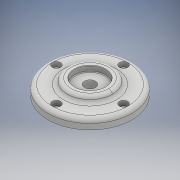
# Autodesk Inventor part: 도면2-3번
Saved by Autodesk Inventor 2018.3 (Build 223284000, 284)
## iProperties
Created: 2019-10-10
Part Number: 도면2-3번
Material: 일반
Document SubType Name: Modeling
Designer: MyTool
Density: 1 g/cm^3
Appearance: 기본값
Author: MyTool
Autodesk Inventor part; units mm, degrees
ref_plane "YZ Plane" through (0, 0, 0) normal (1, 0, 0) x (0, 1, 0)
ref_plane "XZ Plane" through (0, 0, 0) normal (0, 1, 0) x (-1, 0, 0)
ref_plane "XY Plane" through (0, 0, 0) normal (0, 0, 1) x (1, 0, 0)
sketch "스케치4" plane through (0, 0, 0) normal (0, 0, 1) x (1, 0, 0)
  circle A0 centre (0, 0) radius 30
  dimension "d28" = 60
  constraints: 1 centre point, 1 coincident
  measures "d28" diameter of A0
extrude "돌출4" add sketch "스케치4" along normal blind 7
sketch "스케치5" plane through (0, 0, 7) normal (0, 0, 1) x (1, 0, 0)
  circle A0 centre (0, 0) radius 16
  dimension "d31" = 32
  constraints: 1 centre point, 1 coincident
  measures "d31" diameter of A0
extrude "돌출5" add sketch "스케치5" along normal blind 4
sketch "스케치6" plane through (0, 0, 0) normal (0, 0, -1) x (-1, 0, 0)
  circle A0 centre (0, 0) radius 17.5
  dimension "d34" = 35
  constraints: 1 centre point, 1 coincident
  measures "d34" diameter of A0
extrude "돌출6" add sketch "스케치6" along normal blind 4
sketch "스케치8" plane through (0, 0, 11) normal (0, 0, 1) x (1, 0, 0)
  circle A0 centre (0, 0) radius 11
  dimension "d41" = 22
  constraints: 1 centre point, 1 coincident
  measures "d41" diameter of A0
extrude "돌출8" cut sketch "스케치8" against normal blind 4
sketch "스케치9" plane through (0, 0, -4) normal (0, 0, -1) x (-1, 0, 0)
  circle A0 centre (0, 0) radius 9.5
  dimension "d44" = 19
  constraints: 1 centre point, 1 coincident
  measures "d44" diameter of A0
extrude "돌출9" cut sketch "스케치9" against normal blind 4
sketch "스케치11" plane through (0, 0, 7) normal (0, 0, 1) x (1, 0, 0)
  circle A0 centre (0, 0) radius 4
  dimension "d49" = 8
  constraints: 1 centre point, 1 coincident
  measures "d49" diameter of A0
extrude "돌출10" cut sketch "스케치11" against normal up to next
sketch "스케치12" plane through (0, 0, 7) normal (0, 0, 1) x (1, 0, 0)
  circle A0 centre (0, 24) radius 3
  point P0 (0, 0)
  dimension "d61" = 6
  dimension "d62" = 24
  constraints: 1 centre point
  measures "d61" diameter of A0
  measures "d62" distance of point (0, 0) A0.centre
hole "구멍1" at (0, 24, 7) direction (0, 0, -1) diameter 3.4 end through all counterbore diameter 6 counterbore depth 3.3
pattern_circular "원형 패턴2" count 4 over 360 about axis through (0, 0, 7) along (0, 0, -1) of "구멍1"
fillet "모깎기3" radius 3 3 edges at (-30, 0, 7) (-16, 0, 7) (-16, 0, 11)
chamfer "모따기5" distance 1 angle 45 1 edges at (17.5, 0, -4)
chamfer "모따기6" distance 0.4 angle 30 1 edges at (-11, 0, 11) measured on face at (10.9643, -0.8851, 8.3333)
fillet "모깎기4" radius 0.5 1 edges at (-11, 0, 7)
